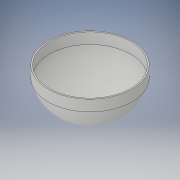
# Autodesk Inventor part: bottom_shell_v2
Saved by Autodesk Inventor 2018 (Build 220112000, 112)
## iProperties
Created: 2018-03-20
Part Number: bottom_shell_v2
Material: Generic
Document SubType Name: Modeling
Designer: scwu
Density: 1 g/cm^3
Appearance: Default
Author: scwu
Autodesk Inventor part; units mm, degrees
ref_plane "YZ Plane" through (0, 0, 0) normal (1, 0, 0) x (0, 1, 0)
ref_plane "XZ Plane" through (0, 0, 0) normal (0, 1, 0) x (-1, 0, 0)
ref_plane "XY Plane" through (0, 0, 0) normal (0, 0, 1) x (1, 0, 0)
sketch "Sketch1" plane through (0, 0, 0) normal (0, 0, 1) x (1, 0, 0)
  arc A0 (-82.1906, -22.0229) -> (0, -85.09) centre (0, 0) ccw
  line L0 (0, 0) -> (-82.1906, -22.0229) construction
  line L1 (0, 0) -> (0, -85.09) construction
  line L2 (-82.1906, -22.0229) -> (-82.1906, 0)
  line L3 (-82.1906, 0) -> (0, 0)
  line L4 (0, -85.09) -> (0, 0)
  dimension "d0" = 85.09
  dimension "d2" = 75
  constraints: 10 end point, 2 perpendicular, 2 point on circle, 1 centre point, 1 coincident, 1 vertical
  measures "d0" radius of A0
  measures "d2" angle of L0 L1
revolve "Revolution1" add sketch "Sketch1" angle 360 about axis through (0, 0, 0) along (0, -1, 0)
shell "Shell1" thickness 2.54 outward yes removed faces 1 at (10.8076, 0, -35.4243)
body "Solid1"
